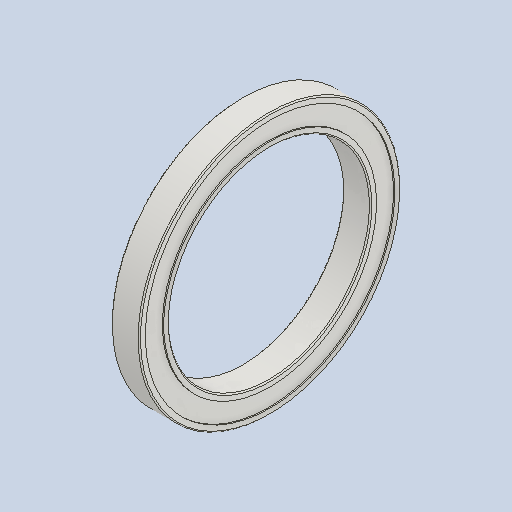
# Autodesk Inventor part: C-E6810ZZ
Saved by Autodesk Inventor 2025.3 (Build 293356030, 356C)
## iProperties
Category: PARTsolutions
Company: MISUMI
Created: 2025-09-20
Part Number: C-E6810ZZ
Material: 강철, 가공됨
Catalog Web Link: www.cadenas.de
Description: C-E6___ZZ-Economy Deep Groove Ball Bearing - Double Shielded, Single Row
Vendor: MISUMI
Document SubType Name: Modeling
Designer: psAdmin
Manufacturer: MISUMI
Mass: 70.1858 g
Surface Area: 53.7803 cm^2
Volume: 8.94087 cm^3
Density: 7.85 g/cm^3
Appearance: 강철
PSOL_IDENT_0: {$CADENAS_DATA/23d-libs/misumi/metric/12_bearing_holders/c_e6700zz.prj},162 {VTYP=3D},{NB=C-E6810ZZ}
PSOL_IDENT_1: ,{LINA=C-E6810ZZ},{NN=C-E6___ZZ},{DATE=29.05.2023 02:13:12},{GEOMDATE=25.05.2021 01:16:58},{VERSION=
PSOL_IDENT_2: },{LINEID=350},{WBVAR=},{WBNUMERIC=}  {NB=C-E6810ZZ},{LINA=C-E6810ZZ},{KT=DUMMY},{PN=C-E6810ZZ},{TS=
PSOL_IDENT_3: C-E6810ZZ},{DD=50},{D=65},{B=7},{RR=0.3},{AA=6.3560},{BB=1.5000},{CC=1.4500}
NB: C-E6810ZZ
NN: C-E6___ZZ
NT: Economy Deep Groove Ball Bearing - Double Shielded, Single Row
NBSYN: $PN.
LINA: C-E6810ZZ
CATALOG: Misumi
PN: C-E6810ZZ
TS: C-E6810ZZ
DD: 50
D: 65
B: 7
RR: 0.3
SUPPLIER: MISUMI
ARTICLENO: C-E6810ZZ
BOMINFO: C-E6810ZZ
CREATOR: CADENAS GmbH
Title: C-E6810ZZ
Author: Cadenas PARTsolutions
Comments: Economy Deep Groove Ball Bearing - Double Shielded, Single Row
Autodesk Inventor part; units mm, degrees
sketch "Sketch_1" plane through (0, 0, 0) normal (0, 0, 1) x (1, 0, 0)
  line L0 (7, 0) -> (0, 0)
  arc A0 (0, 25.3) -> (0.3, 25) centre (0.3, 25.3) ccw
  line L1 (0.3, 25) -> (6.7, 25)
  arc A1 (6.7, 25) -> (7, 25.3) centre (6.7, 25.3) ccw
  line L2 (7, 25.3) -> (7, 26.45)
  line L3 (7, 26.45) -> (6.678, 26.45)
  line L4 (6.678, 26.45) -> (6.678, 31)
  line L5 (6.678, 31) -> (7, 31)
  line L6 (7, 31) -> (7, 32.2)
  arc A2 (7, 32.2) -> (6.7, 32.5) centre (6.7, 32.2) ccw
  line L7 (6.7, 32.5) -> (0.3, 32.5)
  arc A3 (0.3, 32.5) -> (0, 32.2) centre (0.3, 32.2) ccw
  line L8 (0, 32.2) -> (0, 31)
  line L9 (0, 31) -> (0.322, 31)
  line L10 (0.322, 31) -> (0.322, 26.45)
  line L11 (0.322, 26.45) -> (0, 26.45)
  line L12 (0, 26.45) -> (0, 25.3)
  constraints: 26 end point, 8 point on circle, 4 centre point
revolve "Revolution1" add sketch "Sketch_1" angle 360 about axis through (7, 0, 0) along (1, 0, 0)
ref_plane "center_point_XY" through (3.5, 0, 0) normal (1, 0, 0) x (0, 0, -1)
ref_plane "center_point_YZ" through (3.5, 0, 0) normal (0, 0, -1) x (0, 1, 0)
ref_plane "center_point_ZX" through (3.5, 0, 0) normal (0, 1, 0) x (1, 0, 0)
ref_plane "to_housing_XY" through (0, 0, 0) normal (1, 0, 0) x (0, 0, -1)
ref_plane "to_housing_YZ" through (0, 0, 0) normal (0, 0, -1) x (0, 1, 0)
ref_plane "to_housing_ZX" through (0, 0, 0) normal (0, 1, 0) x (1, 0, 0)
ref_plane "to_ring_XY" through (6.356, 0, 0) normal (1, 0, 0) x (0, 0, -1)
ref_plane "to_ring_YZ" through (6.356, 0, 0) normal (0, 0, -1) x (0, 1, 0)
ref_plane "to_ring_ZX" through (6.356, 0, 0) normal (0, 1, 0) x (1, 0, 0)
body "Solid1"
